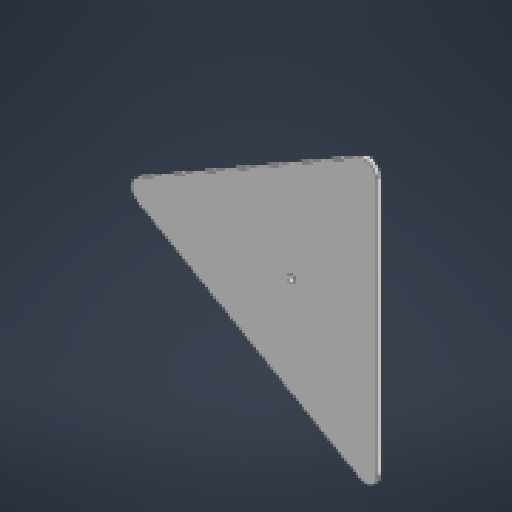
# Autodesk Inventor part: multifunctional_lvl
Saved by Autodesk Inventor 2024 (Build 280153000, 153)
## iProperties
Created: 2026-03-28
Part Number: multifunctional_lvl
Material: Generic
Document SubType Name: Modeling
Designer: schar
Density: 1 g/cm^3
Appearance: Default
Author: schar
Autodesk Inventor part; units mm, degrees
ref_plane "YZ Plane" through (0, 0, 0) normal (1, 0, 0) x (0, 1, 0)
ref_plane "XZ Plane" through (0, 0, 0) normal (0, 1, 0) x (-1, 0, 0)
ref_plane "XY Plane" through (0, 0, 0) normal (0, 0, 1) x (1, 0, 0)
sketch "Sketch1" plane through (0, 0, 0) normal (0, 0, 1) x (1, 0, 0)
  line L0 (-154.4076, 199.4033) -> (65.098, -180.7915)
  circle A0 centre (-39.282, 0) radius 2.75
  circle A1 centre (15, 94.0192) radius 8.5
  circle A2 centre (-147.8461, 0) radius 8.5
  circle A3 centre (15, -94.0192) radius 8.5
  line L1 (15, 94.0192) -> (15, -94.0192)
  line L2 (15, -94.0192) -> (-147.8461, 0)
  line L3 (-147.8461, 0) -> (15, 94.0192)
  line L4 (53.7758, 126.2214) -> (-193.87, -16.757)
  line L5 (23.5, -175.7783) -> (23.5, 120.7175)
  line L6 (64.2969, -132.2958) -> (-207.0406, 24.361)
  circle A4 centre (-39.282, 0) radius 2.75
  circle A5 centre (-39.282, 0) radius 2.5 projected
  point P0 (0, 0)
  point P1 (23.5, -94.0192)
  point P2 (23.5, 94.0192)
  point P3 (10.75, 101.3805)
  point P4 (-152.0961, 7.3612)
  point P5 (-152.0961, -7.3612)
  point P6 (10.75, -101.3805)
  dimension "d2" = 17
  dimension "d3" = 360
  dimension "d4" = 5.5
  constraints: 14 end point, 6 tangent, 5 centre point, 5 coincident, 14 other
  measures "d2" diameter of A1
  measures "d4" diameter of A4
extrude "Extrusion1" add sketch "Sketch1" along normal blind 3 contours L4 A1 L3 L0 | L0 L3 A2 L4 | L3 A1 L1 A3 L0 A0 | L0 A0 A3 L2 A2 L3 | A1 L1 L3 | A2 L3 L2 | A2 L2 L3 | L3 L1 A1 | L5 A3 L1 A1 | A2 L2 A3 L6 | A3 L0 L1 | A3 L2 L0 | A3 L1 L0 | L0 L2 A3
sketch "Sketch2" plane through (0, 0, 3) normal (0, 0, 1) x (1, 0, 0)
  circle A0 centre (-147.8461, 0) radius 2.5 projected
  circle A1 centre (15, 94.0192) radius 2.5 projected
  circle A2 centre (15, -94.0192) radius 2.5 projected
  line L0 (-152.0961, -7.3612) -> (10.75, -101.3805) projected
  line L1 (10.75, 101.3805) -> (-152.0961, 7.3612) projected
  point P0 (0, 0)
extrude "Extrusion2" cut sketch "Sketch2" against normal blind 3
sketch "Sketch3" plane through (0, 0, 3) normal (0, 0, 1) x (1, 0, 0)
  circle A0 centre (-39.282, 0) radius 2.75 projected
  line L0 (-39.282, 0) -> (-59.282, 0)
  line L1 (-59.282, 0) -> (-79.282, 0)
  line L2 (-79.282, 0) -> (-94.282, 0)
  line L3 (-94.282, 0) -> (-109.282, 0)
  line L4 (-59.282, 0) -> (-49.282, 17.3205)
  line L5 (-49.282, 17.3205) -> (-29.282, 17.3205)
  line L6 (-29.282, 17.3205) -> (-19.282, 0)
  line L7 (-19.282, 0) -> (-29.282, -17.3205)
  line L8 (-29.282, -17.3205) -> (-49.282, -17.3205)
  line L9 (-49.282, -17.3205) -> (-59.282, 0)
  line L10 (-79.282, 0) -> (-59.282, 34.641)
  line L11 (-59.282, 34.641) -> (-19.282, 34.641)
  line L12 (-19.282, 34.641) -> (0.718, 0)
  line L13 (0.718, 0) -> (-19.282, -34.641)
  line L14 (-19.282, -34.641) -> (-59.282, -34.641)
  line L15 (-59.282, -34.641) -> (-79.282, 0)
  line L16 (-94.282, 0) -> (-66.782, 47.6314)
  line L17 (-66.782, 47.6314) -> (-11.782, 47.6314)
  line L18 (-11.782, 47.6314) -> (15.718, 0)
  line L19 (15.718, 0) -> (-11.782, -47.6314)
  line L20 (-11.782, -47.6314) -> (-66.782, -47.6314)
  line L21 (-66.782, -47.6314) -> (-94.282, 0)
  circle A1 centre (-49.282, -17.3205) radius 2.5
  circle A2 centre (-59.282, -34.641) radius 2.5
  circle A3 centre (-66.782, -47.6314) radius 2.5
  circle A4 centre (-29.282, -17.3205) radius 2.5
  circle A5 centre (-19.282, -34.641) radius 2.5
  circle A6 centre (-11.782, -47.6314) radius 2.5
  circle A7 centre (-19.282, 0) radius 2.5
  circle A8 centre (0.718, 0) radius 2.5
  circle A9 centre (15.718, 0) radius 2.5
  circle A10 centre (-29.282, 17.3205) radius 2.5
  circle A11 centre (-19.282, 34.641) radius 2.5
  circle A12 centre (-11.782, 47.6314) radius 2.5
  circle A13 centre (-49.282, 17.3205) radius 2.5
  circle A14 centre (-59.282, 34.641) radius 2.5
  circle A15 centre (-66.782, 47.6314) radius 2.5
  circle A16 centre (-59.282, 0) radius 2.5
  circle A17 centre (-79.282, 0) radius 2.5
  circle A18 centre (-94.282, 0) radius 2.5
  line L22 (-19.282, -34.641) -> (-11.782, -47.6314)
  line L23 (-11.782, -47.6314) -> (-1.782, -64.9519)
  line L24 (-1.782, -64.9519) -> (8.218, -82.2724)
  circle A19 centre (-1.782, -64.9519) radius 2.5
  circle A20 centre (8.218, -82.2724) radius 2.5
  circle A21 centre (-1.782, 64.9519) radius 2.5
  circle A22 centre (8.218, 82.2724) radius 2.5
  circle A23 centre (-114.282, 0) radius 2.5
  circle A24 centre (-134.282, 0) radius 2.5
  line L25 (-80.532, 23.8157) -> (-39.282, 0)
  line L26 (-39.282, 0) -> (-39.282, 47.6314)
  line L27 (-39.282, 0) -> (1.968, 23.8157)
  line L28 (-39.282, 0) -> (1.968, -23.8157)
  line L29 (-39.282, 0) -> (-39.282, -47.6314)
  line L30 (-39.282, 0) -> (-80.532, -23.8157)
  circle A25 centre (-80.532, -23.8157) radius 7.5
  circle A26 centre (-39.282, -47.6314) radius 7.5
  circle A27 centre (1.968, -23.8157) radius 7.5
  circle A28 centre (1.968, 23.8157) radius 7.5
  circle A29 centre (-39.282, 47.6314) radius 7.5
  circle A30 centre (-80.532, 23.8157) radius 7.5
  point P0 (0, 0)
  dimension "d9" = 20
  dimension "d10" = 20
  dimension "d11" = 15
  dimension "d12" = 15
  dimension "d13" = 5
  dimension "d14" = 5
  dimension "d15" = 5
  dimension "d18" = 360
  dimension "d20" = 20
  dimension "d21" = 20
  dimension "d22" = 5
  dimension "d23" = 5
  dimension "d24" = 17.3205
  dimension "d27" = 360
  dimension "d31" = 15
  dimension "d32" = 15
  dimension "d33" = 15
  dimension "d34" = 15
  dimension "d35" = 15
  dimension "d36" = 15
  constraints: 62 end point, 30 centre point, 14 coincident, 6 midpoint, 4 point on line, 2 collinear, 1 horizontal, 89 other
  measures "d9" distance of L0.start L0.end
  measures "d10" distance of L0.end L1.end
  measures "d11" distance of L1.end L2.end
  measures "d12" distance of L2.end L3.end
  measures "d13" diameter of A1
  measures "d14" diameter of A2
  measures "d15" diameter of A3
  measures "d20" distance of L22.end L23.end
  measures "d21" distance of L23.end L24.end
  measures "d22" diameter of A19
  measures "d23" diameter of A20
  measures "d24" distance from line of A19.centre L20
  measures "d31" diameter of A25
  measures "d32" diameter of A26
  measures "d33" diameter of A27
  measures "d34" diameter of A28
  measures "d35" diameter of A29
  measures "d36" diameter of A30
extrude "Extrusion3" cut sketch "Sketch3" against normal blind 3 contours A10 L5 L6 | L6 L5 A10 | A7 L7 L6 | L6 L7 A7 | A4 L8 L7 | L7 L8 A4 | A13 L4 L5 | L5 L4 A13 | A16 L9 L0 | L0 L4 A16 | A11 L11 L12 | L12 L11 A11 | A8 L13 L12 | L12 L13 A8 | A28 L18 L27 | L27 L18 A28 | A1 L9 L8 | L8 L9 A1 | A5 L22 L13 | L13 L14 A5 | A27 L19 L28 | L28 L19 A27 | L4 L1 A16 | A14 L10 L11 | L11 L10 A14 | A29 L17 L26 | L26 L17 A29 | L9 A16 L1 | L18 A28 | A20 | A19 L24 L23 | L23 L24 A19 | L14 L22 A5 | A2 L15 L14 | L14 L15 A2 | A26 L20 L29 | L29 L20 A26 | L19 A27 | A17 L1 L10 | L10 L2 A17 | A30 L16 L25 | L25 L16 A30 | L17 A29 | A17 L2 L15 | L15 L1 A17 | A25 L21 L30 | L30 L21 A25 | A12 L17 L18 | L18 L17 A12 | A9 L19 L18 | L18 L19 A9 | L20 A26 | A6 L23 L19 | L19 L22 A6 | L16 A30 | A15 L16 L17 | L17 L16 A15 | L21 A25 | L22 L20 A6 | L20 L23 A6 | A3 L21 L20 | L20 L21 A3 | A18 L21 L2 | L2 L16 A18 | L16 L3 A18 | A18 L3 L21 | A21 | A22 | A23 | A24
body "Solid1"
